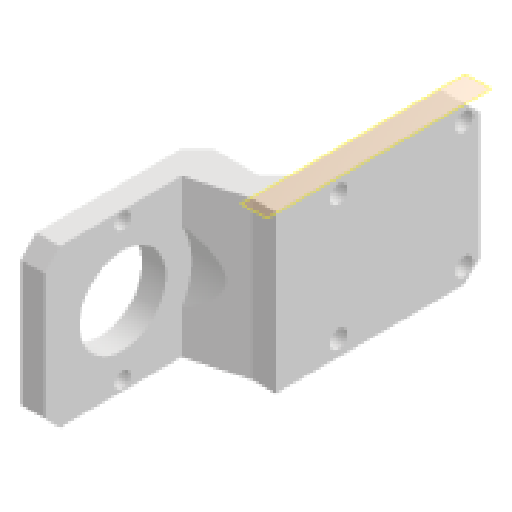
# Autodesk Inventor part: 40_XYZstage_micrometer_motorized_nema8_samplemount_lightsheet_screwed
Saved by Autodesk Inventor 2024.1 (Build 281209000, 209)
## iProperties
Created: 2024-03-17
Part Number: 40_XYZstage_micrometer_motorized_nema8_samplemount_lightsheet_screwed
Material: Generisch
Document SubType Name: Modeling
Designer: diederichbenedict
Density: 1 g/cm^3
Appearance: Vorgabe
Author: diederichbenedict
Autodesk Inventor part; units mm, degrees
ref_plane "YZ Plane" through (0, 0, 0) normal (1, 0, 0) x (0, 1, 0)
ref_plane "XZ Plane" through (0, 0, 0) normal (0, 1, 0) x (-1, 0, 0)
ref_plane "XY Plane" through (0, 0, 0) normal (0, 0, 1) x (1, 0, 0)
sketch "Skizze1" plane through (0, 0, 0) normal (1, 0, 0) x (0, 1, 0)
  line L0 (-20, -20) -> (20, -20)
  line L1 (20, -20) -> (20, 20)
  line L2 (20, 20) -> (-20, 20)
  line L3 (-20, 20) -> (-20, -20)
  line L4 (-20, -20) -> (20, 20) construction
  line L5 (20, -20) -> (-20, 20) construction
  line L6 (-16, -16) -> (16, -16) construction
  line L7 (16, -16) -> (16, 16) construction
  line L8 (16, 16) -> (-16, 16) construction
  line L9 (-16, 16) -> (-16, -16) construction
  line L10 (-16, -16) -> (16, 16) construction
  line L11 (16, -16) -> (-16, 16) construction
  circle A0 centre (16, 16) radius 2.25
  circle A1 centre (16, -16) radius 2.25
  circle A2 centre (-16, -16) radius 2.25
  circle A3 centre (-16, 16) radius 2.25
  line L12 (-20, 20) -> (-32, 20)
  line L13 (-32, 20) -> (-32, -20)
  line L14 (-32, -20) -> (-20, -20)
  line L15 (-20, -20) -> (-20, 20)
  point P0 (0, 0)
  dimension "d0" = 40
  dimension "d1" = 40
  dimension "d2" = 32
  dimension "d3" = 32
  dimension "d4" = 4.5
  dimension "d5" = 4.5
  dimension "d6" = 4.5
  dimension "d7" = 4.5
  dimension "d8" = 12
  constraints: 32 end point, 6 parallel, 4 centre point, 4 coincident, 4 midpoint, 3 horizontal, 3 perpendicular
  measures "d0" distance of L2.end L1.end
  measures "d1" distance of L1.end L0.end
  measures "d2" distance of L8.end L7.end
  measures "d3" distance of L7.end L6.end
  measures "d4" diameter of A0
  measures "d5" diameter of A1
  measures "d6" diameter of A2
  measures "d7" diameter of A3
  measures "d8" distance of L14.end L13.end
extrude "Extrusion1" add sketch "Skizze1" along normal blind 6
ref_plane "Arbeitsebene1" through (0, -32, 20) normal (0, 0, 1) x (1, 0, 0)
sketch "Skizze2" plane through (0, -32, 20) normal (0, 0, 1) x (1, 0, 0)
  line L0 (0, 52) -> (0, 0) projected
  line L1 (0, 0) -> (6, 0) projected
  line L2 (6, 52) -> (6, 0) projected
  line L3 (0, 52) -> (6, 52) projected
  line L4 (-20, 6) -> (-14, 6)
  line L5 (-14, 6) -> (-14, -39)
  line L6 (-14, -39) -> (-20, -39)
  line L7 (-20, -39) -> (-20, 6)
  line L8 (0, 0) -> (-14, -4)
  line L9 (-14, 6) -> (0, 6)
  point P0 (0, 32)
  point P1 (-17, -39)
  point P2 (-17, 6)
  dimension "d12" = 6
  dimension "d13" = 45
  dimension "d14" = 6
  dimension "d15" = 14
  dimension "d16" = 10
  constraints: 12 end point, 2 midpoint, 2 parallel, 2 perpendicular, 2 point on line, 1 horizontal
  measures "d12" distance of L5.end L6.end
  measures "d13" distance of point (-17, -39) point (-17, 6)
  measures "d14" distance from line of point (-17, 6) L1
  measures "d15" distance between parallel lines of L0 L5
  measures "d16" vertical distance of L8.end point (-17, 6)
extrude "Extrusion2" add sketch "Skizze2" against normal up to surface (40 mm away) contours L0 L8 L5 L9 | L5 L6 L7 L4
chamfer "Fasen1" distance 4 angle 45 6 edges at (-20, -26, 0) (0, -26, 0) (-17, -71, -20) (-17, -71, 20) (3, 20, -20) (3, 20, 20)
sketch "Skizze3" plane through (-14, -36, 20) normal (1, 0, 0) x (0, 0, -1)
  line L0 (4, -35) -> (0, -31) projected
  line L1 (4, -35) -> (36, -35) projected
  line L2 (40, -31) -> (36, -35) projected
  line L3 (40, 0) -> (40, -31) projected
  line L4 (0, 0) -> (40, 0) projected
  line L5 (0, -31) -> (0, 0) projected
  circle A0 centre (20, -15) radius 20
  circle A1 centre (20, -15) radius 17.5
  point P0 (20, 36)
  dimension "d22" = 35
  constraints: 3 tangent, 2 centre point, 1 coincident
  measures "d22" diameter of A1
extrude "Extrusion3" cut sketch "Skizze3" along normal through all contours A1 L4 | L4 A1
sketch "Skizze4" plane through (-14, -67, 20) normal (1, 0, 0) x (0, 0, -1)
  line L0 (0, 31) -> (10.9861, 31) projected
  line L1 (0, 0) -> (0, 31) projected
  line L2 (4, -4) -> (0, 0) projected
  line L3 (4, -4) -> (36, -4) projected
  line L4 (40, 0) -> (36, -4) projected
  line L5 (40, 31) -> (40, 0) projected
  line L6 (29.0139, 31) -> (40, 31) projected
  arc A0 (29.0139, 31) -> (10.9861, 31) centre (20, 16) ccw projected
  circle A1 centre (20, 16) radius 17.5
  circle A2 centre (2.5, 16) radius 2
  circle A3 centre (37.5, 16) radius 2
  point P0 (20, 67)
  dimension "d25" = 4
  dimension "d26" = 4
  constraints: 3 centre point, 3 coincident, 2 point on circle, 1 concentric
  measures "d25" diameter of A2
  measures "d26" diameter of A3
extrude "Extrusion4" cut sketch "Skizze4" against normal blind 10 contours A2 A1 | A1 A2 | A3 A1 | A1 A3
sketch "Skizze5" plane through (-14, -67, 20) normal (1, 0, 0) x (0, 0, -1)
  arc A0 (29.0139, 31) -> (10.9861, 31) centre (20, 16) ccw projected
  line L0 (0, 35) -> (40, 35) projected
  line L1 (0, 31) -> (0, 35) projected
  line L2 (0, 31) -> (10.9861, 31) projected
  circle A1 centre (20, 16) radius 11
  line L3 (29.0139, 31) -> (40, 31) projected
  line L4 (40, 35) -> (40, 31) projected
  point P0 (20, 67)
  dimension "d29" = 22
  constraints: 1 centre point, 1 coincident
  measures "d29" diameter of A1
extrude "Extrusion5" cut sketch "Skizze5" against normal blind 10 contours A1
